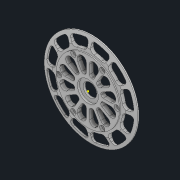
# Autodesk Inventor part: taiko_01
Saved by Autodesk Inventor 2022 (Build 260153000, 153)
## iProperties
Created: 2024-06-02
Part Number: taiko_01
Material: 一般
Document SubType Name: Modeling
Designer: gisen
Density: 1 g/cm^3
Appearance: 既定
Author: gisen
Autodesk Inventor part; units mm, degrees
ref_plane "YZ Plane" through (0, 0, 0) normal (1, 0, 0) x (0, 1, 0)
ref_plane "XZ Plane" through (0, 0, 0) normal (0, 1, 0) x (-1, 0, 0)
ref_plane "XY Plane" through (0, 0, 0) normal (0, 0, 1) x (1, 0, 0)
sketch "スケッチ1" plane through (0, 0, 0) normal (0, 0, 1) x (1, 0, 0)
  circle A0 centre (0, 0) radius 45
  circle A1 centre (0, 0) radius 6.5
  dimension "d0" = 90
  dimension "d9" = 13
  constraints: 2 centre point, 2 coincident
  measures "d0" diameter of A0
  measures "d9" diameter of A1
extrude "押し出し1" add sketch "スケッチ1" along normal blind 4
sketch "スケッチ2" plane through (0, 0, 4) normal (0, 0, 1) x (1, 0, 0)
  circle A0 centre (0, 0) radius 45 projected
  circle A1 centre (0, 0) radius 30.4
  dimension "d3" = 60.8
  constraints: 1 centre point, 1 coincident
  measures "d3" diameter of A1
extrude "押し出し2" cut sketch "スケッチ2" against normal blind 1
chamfer "面取り1" distance 2 distance2 10 1 edges at (-45, 0, 3) measured on face at (39.7326, -21.1262, 2)
sketch "スケッチ3" plane through (0, 0, 4) normal (0, 0, 1) x (1, 0, 0)
  circle A0 centre (0, 0) radius 10.05
  dimension "d10" = 20.1
  constraints: 1 centre point, 1 coincident
  measures "d10" diameter of A0
extrude "押し出し3" cut sketch "スケッチ3" against normal blind 2
sketch "スケッチ4" plane through (0, 0, 4) normal (0, 0, 1) x (1, 0, 0)
  circle A0 centre (0, 0) radius 45 construction
  circle A1 centre (0, 0) radius 30.4 construction
  circle A2 centre (0, 0) radius 10.05 construction
  circle A3 centre (0, 0) radius 13.05 construction
  circle A4 centre (0, 0) radius 42 construction
  circle A5 centre (0, 0) radius 32.5 construction
  line L0 (0, 0) -> (-45, 0) construction
  circle A6 centre (0, 0) radius 27.75 construction
  circle A7 centre (-27.75, 0) radius 4 construction
  line L1 (0, -1.5) -> (-45, -1.5) construction
  line L2 (-45, -1.5) -> (-45, 1.5) construction
  line L3 (-45, 1.5) -> (0, 1.5) construction
  line L4 (0, 1.5) -> (0, -1.5) construction
  circle A8 centre (-27.75, 0) radius 1.25
  line L5 (0.75, -1.299) -> (-38.2211, -23.799) construction
  line L6 (-39.7211, -21.201) -> (-0.75, 1.299) construction
  line L7 (1.299, -0.75) -> (-21.201, -39.7211) construction
  line L8 (-23.799, -38.2211) -> (-1.299, 0.75) construction
  line L9 (1.5, 0) -> (1.5, -45) construction
  line L10 (-1.5, -45) -> (-1.5, 0) construction
  line L11 (1.299, 0.75) -> (23.799, -38.2211) construction
  line L12 (21.201, -39.7211) -> (-1.299, -0.75) construction
  line L13 (0.75, 1.299) -> (39.7211, -21.201) construction
  line L14 (38.2211, -23.799) -> (-0.75, -1.299) construction
  line L15 (0, 1.5) -> (45, 1.5) construction
  line L16 (45, -1.5) -> (0, -1.5) construction
  line L17 (-0.75, 1.299) -> (38.2211, 23.799) construction
  line L18 (39.7211, 21.201) -> (0.75, -1.299) construction
  line L19 (-1.299, 0.75) -> (21.201, 39.7211) construction
  line L20 (23.799, 38.2211) -> (1.299, -0.75) construction
  line L21 (-1.5, 0) -> (-1.5, 45) construction
  line L22 (1.5, 45) -> (1.5, 0) construction
  line L23 (-1.299, -0.75) -> (-23.799, 38.2211) construction
  line L24 (-21.201, 39.7211) -> (1.299, 0.75) construction
  line L25 (-0.75, -1.299) -> (-39.7211, 21.201) construction
  line L26 (-38.2211, 23.799) -> (0.75, 1.299) construction
  circle A9 centre (-13.875, -24.0322) radius 4 construction
  circle A10 centre (-13.875, -24.0322) radius 1.25
  circle A11 centre (13.875, -24.0322) radius 4 construction
  circle A12 centre (13.875, -24.0322) radius 1.25
  circle A13 centre (27.75, 0) radius 4 construction
  circle A14 centre (27.75, 0) radius 1.25
  circle A15 centre (13.875, 24.0322) radius 4 construction
  circle A16 centre (13.875, 24.0322) radius 1.25
  circle A17 centre (-13.875, 24.0322) radius 4 construction
  circle A18 centre (-13.875, 24.0322) radius 1.25
  arc A19 (-12.9635, -1.5) -> (-11.9767, -5.1827) centre (0, 0) ccw
  arc A20 (-10.4767, -7.7808) -> (-7.7808, -10.4767) centre (0, 0) ccw
  arc A21 (-23.2471, -15.1538) -> (-17.1859, -21.7877) centre (0, 0) ccw
  arc A22 (-27.4617, -3.9896) -> (-24.7471, -12.5557) centre (0, 0) ccw
  arc A23 (-27.3658, -17.5317) -> (-17.5317, -27.3658) centre (0, 0) ccw
  arc A24 (-32.4654, -1.5) -> (-28.8658, -14.9336) centre (0, 0) ccw
  arc A25 (-27.4617, -3.9896) -> (-24.0419, -1.5) centre (-27.75, 0) ccw
  arc A26 (-13.32, -20.0709) -> (-17.1859, -21.7877) centre (-13.875, -24.0322) ccw
  arc A27 (-41.9732, -1.5) -> (-37.0999, -19.6876) centre (0, 0) ccw
  arc A28 (-35.5999, -22.2856) -> (-22.2856, -35.5999) centre (0, 0) ccw
  line L27 (-7.7808, -10.4767) -> (-13.32, -20.0709)
  line L28 (-17.5317, -27.3658) -> (-22.2856, -35.5999)
  line L29 (-27.3658, -17.5317) -> (-35.5999, -22.2856)
  line L30 (-10.4767, -7.7808) -> (-23.2471, -15.1538)
  line L31 (-11.9767, -5.1827) -> (-24.7471, -12.5557)
  line L32 (-28.8658, -14.9336) -> (-37.0999, -19.6876)
  line L33 (-12.9635, -1.5) -> (-24.0419, -1.5)
  line L34 (-32.4654, -1.5) -> (-41.9732, -1.5)
  line L35 (5.1827, -11.9767) -> (10.7219, -21.5709)
  arc A29 (10.7219, -21.5709) -> (10.2758, -25.7773) centre (13.875, -24.0322) ccw
  arc A30 (1.5, -27.7094) -> (10.2758, -25.7773) centre (0, 0) ccw
  arc A31 (1.5, -12.9635) -> (5.1827, -11.9767) centre (0, 0) ccw
  line L36 (1.5, -12.9635) -> (1.5, -27.7094)
  line L37 (-1.5, -12.9635) -> (-1.5, -27.7094)
  arc A32 (-10.2758, -25.7773) -> (-1.5, -27.7094) centre (0, 0) ccw
  arc A33 (-5.1827, -11.9767) -> (-1.5, -12.9635) centre (0, 0) ccw
  line L38 (-5.1827, -11.9767) -> (-10.7219, -21.5709)
  arc A34 (-10.2758, -25.7773) -> (-10.7219, -21.5709) centre (-13.875, -24.0322) ccw
  arc A35 (-14.9336, -28.8658) -> (-1.5, -32.4654) centre (0, 0) ccw
  line L39 (-14.9336, -28.8658) -> (-19.6876, -37.0999)
  arc A36 (-19.6876, -37.0999) -> (-1.5, -41.9732) centre (0, 0) ccw
  line L40 (-1.5, -32.4654) -> (-1.5, -41.9732)
  line L41 (14.9336, -28.8658) -> (19.6876, -37.0999)
  arc A37 (1.5, -41.9732) -> (19.6876, -37.0999) centre (0, 0) ccw
  arc A38 (1.5, -32.4654) -> (14.9336, -28.8658) centre (0, 0) ccw
  line L42 (1.5, -32.4654) -> (1.5, -41.9732)
  line L43 (12.9635, -1.5) -> (24.0419, -1.5)
  arc A39 (24.0419, -1.5) -> (27.4617, -3.9896) centre (27.75, 0) ccw
  arc A40 (24.7471, -12.5557) -> (27.4617, -3.9896) centre (0, 0) ccw
  arc A41 (11.9767, -5.1827) -> (12.9635, -1.5) centre (0, 0) ccw
  line L44 (11.9767, -5.1827) -> (24.7471, -12.5557)
  line L45 (10.4767, -7.7808) -> (23.2471, -15.1538)
  arc A42 (17.1859, -21.7877) -> (23.2471, -15.1538) centre (0, 0) ccw
  arc A43 (7.7808, -10.4767) -> (10.4767, -7.7808) centre (0, 0) ccw
  line L46 (7.7808, -10.4767) -> (13.32, -20.0709)
  arc A44 (17.1859, -21.7877) -> (13.32, -20.0709) centre (13.875, -24.0322) ccw
  arc A45 (17.5317, -27.3658) -> (27.3658, -17.5317) centre (0, 0) ccw
  line L47 (17.5317, -27.3658) -> (22.2856, -35.5999)
  arc A46 (22.2856, -35.5999) -> (35.5999, -22.2856) centre (0, 0) ccw
  line L48 (27.3658, -17.5317) -> (35.5999, -22.2856)
  line L49 (32.4654, -1.5) -> (41.9732, -1.5)
  arc A47 (37.0999, -19.6876) -> (41.9732, -1.5) centre (0, 0) ccw
  arc A48 (28.8658, -14.9336) -> (32.4654, -1.5) centre (0, 0) ccw
  line L50 (28.8658, -14.9336) -> (37.0999, -19.6876)
  line L51 (7.7808, 10.4767) -> (13.32, 20.0709)
  arc A49 (13.32, 20.0709) -> (17.1859, 21.7877) centre (13.875, 24.0322) ccw
  arc A50 (23.2471, 15.1538) -> (17.1859, 21.7877) centre (0, 0) ccw
  arc A51 (10.4767, 7.7808) -> (7.7808, 10.4767) centre (0, 0) ccw
  line L52 (10.4767, 7.7808) -> (23.2471, 15.1538)
  line L53 (11.9767, 5.1827) -> (24.7471, 12.5557)
  arc A52 (27.4617, 3.9896) -> (24.7471, 12.5557) centre (0, 0) ccw
  arc A53 (12.9635, 1.5) -> (11.9767, 5.1827) centre (0, 0) ccw
  line L54 (12.9635, 1.5) -> (24.0419, 1.5)
  arc A54 (27.4617, 3.9896) -> (24.0419, 1.5) centre (27.75, 0) ccw
  arc A55 (32.4654, 1.5) -> (28.8658, 14.9336) centre (0, 0) ccw
  line L55 (32.4654, 1.5) -> (41.9732, 1.5)
  arc A56 (41.9732, 1.5) -> (37.0999, 19.6876) centre (0, 0) ccw
  line L56 (28.8658, 14.9336) -> (37.0999, 19.6876)
  line L57 (17.5317, 27.3658) -> (22.2856, 35.5999)
  arc A57 (35.5999, 22.2856) -> (22.2856, 35.5999) centre (0, 0) ccw
  arc A58 (27.3658, 17.5317) -> (17.5317, 27.3658) centre (0, 0) ccw
  line L58 (27.3658, 17.5317) -> (35.5999, 22.2856)
  line L59 (-5.1827, 11.9767) -> (-10.7219, 21.5709)
  arc A59 (-10.7219, 21.5709) -> (-10.2758, 25.7773) centre (-13.875, 24.0322) ccw
  arc A60 (-1.5, 27.7094) -> (-10.2758, 25.7773) centre (0, 0) ccw
  arc A61 (-1.5, 12.9635) -> (-5.1827, 11.9767) centre (0, 0) ccw
  line L60 (-1.5, 12.9635) -> (-1.5, 27.7094)
  line L61 (1.5, 12.9635) -> (1.5, 27.7094)
  arc A62 (10.2758, 25.7773) -> (1.5, 27.7094) centre (0, 0) ccw
  arc A63 (5.1827, 11.9767) -> (1.5, 12.9635) centre (0, 0) ccw
  line L62 (5.1827, 11.9767) -> (10.7219, 21.5709)
  arc A64 (10.2758, 25.7773) -> (10.7219, 21.5709) centre (13.875, 24.0322) ccw
  arc A65 (14.9336, 28.8658) -> (1.5, 32.4654) centre (0, 0) ccw
  line L63 (14.9336, 28.8658) -> (19.6876, 37.0999)
  arc A66 (19.6876, 37.0999) -> (1.5, 41.9732) centre (0, 0) ccw
  line L64 (1.5, 32.4654) -> (1.5, 41.9732)
  line L65 (-14.9336, 28.8658) -> (-19.6876, 37.0999)
  arc A67 (-1.5, 41.9732) -> (-19.6876, 37.0999) centre (0, 0) ccw
  arc A68 (-1.5, 32.4654) -> (-14.9336, 28.8658) centre (0, 0) ccw
  line L66 (-1.5, 32.4654) -> (-1.5, 41.9732)
  line L67 (-12.9635, 1.5) -> (-24.0419, 1.5)
  arc A69 (-24.0419, 1.5) -> (-27.4617, 3.9896) centre (-27.75, 0) ccw
  arc A70 (-24.7471, 12.5557) -> (-27.4617, 3.9896) centre (0, 0) ccw
  arc A71 (-11.9767, 5.1827) -> (-12.9635, 1.5) centre (0, 0) ccw
  line L68 (-11.9767, 5.1827) -> (-24.7471, 12.5557)
  line L69 (-10.4767, 7.7808) -> (-23.2471, 15.1538)
  arc A72 (-17.1859, 21.7877) -> (-23.2471, 15.1538) centre (0, 0) ccw
  arc A73 (-7.7808, 10.4767) -> (-10.4767, 7.7808) centre (0, 0) ccw
  line L70 (-7.7808, 10.4767) -> (-13.32, 20.0709)
  arc A74 (-17.1859, 21.7877) -> (-13.32, 20.0709) centre (-13.875, 24.0322) ccw
  arc A75 (-17.5317, 27.3658) -> (-27.3658, 17.5317) centre (0, 0) ccw
  line L71 (-17.5317, 27.3658) -> (-22.2856, 35.5999)
  arc A76 (-22.2856, 35.5999) -> (-35.5999, 22.2856) centre (0, 0) ccw
  line L72 (-27.3658, 17.5317) -> (-35.5999, 22.2856)
  line L73 (-32.4654, 1.5) -> (-41.9732, 1.5)
  arc A77 (-37.0999, 19.6876) -> (-41.9732, 1.5) centre (0, 0) ccw
  arc A78 (-28.8658, 14.9336) -> (-32.4654, 1.5) centre (0, 0) ccw
  line L74 (-28.8658, 14.9336) -> (-37.0999, 19.6876)
  circle A79 centre (-27.75, 0) radius 2.5 construction
  dimension "d14" = 3
  dimension "d15" = 3
  dimension "d16" = 65
  dimension "d17" = 8
  dimension "d18" = 55.5
  dimension "d19" = 3
  dimension "d20" = 2.5
  dimension "d23" = 360
  dimension "d27" = 360
  dimension "d31" = 360
  dimension "d42" = 5
  constraints: 150 end point, 141 point on circle, 77 centre point, 57 coincident, 17 point on line, 6 collinear, 3 parallel, 2 horizontal, 2 midpoint, 1 horizontal alignment, 1 perpendicular, 376 other
  measures "d15" radial gap between concentric circles of A3 A2
  measures "d16" diameter of A5
  measures "d17" diameter of A7
  measures "d18" diameter of A6
  measures "d19" distance between parallel lines of L3 L1
  measures "d20" diameter of A8
  measures "d42" diameter of A79
extrude "押し出し4" cut sketch "スケッチ4" against normal through all
fillet "フィレット1" radius 4 24 edges at (1.5, -32.4654, 1.5) (14.9336, -28.8658, 1.5) (17.5317, -27.3658, 1.5) (27.3658, -17.5317, 1.5) (28.8658, -14.9336, 1.5) (32.4654, -1.5, 1.5) (32.4654, 1.5, 1.5) (28.8658, 14.9336, 1.5) (27.3658, 17.5317, 1.5) (17.5317, 27.3658, 1.5) (14.9336, 28.8658, 1.5) (1.5, 32.4654, 1.5) (-1.5, 32.4654, 1.5) (-14.9336, 28.8658, 1.5) (-17.5317, 27.3658, 1.5) (-27.3658, 17.5317, 1.5) (-28.8658, 14.9336, 1.5) (-32.4654, 1.5, 1.5) (-32.4654, -1.5, 1.5) (-28.8658, -14.9336, 1.5) (-27.3658, -17.5317, 1.5) (-17.5317, -27.3658, 1.5) (-14.9336, -28.8658, 1.5) (-1.5, -32.4654, 1.5)
fillet "フィレット2" radius 4 36 edges at (10.2758, -25.7773, 2) (10.7219, -21.5709, 2) (1.5, -27.7094, 2) (13.32, -20.0709, 2) (17.1859, -21.7877, 2) (23.2471, -15.1538, 2) (24.7471, -12.5557, 2) (27.4617, -3.9896, 2) (24.0419, -1.5, 2) (24.0419, 1.5, 2) (27.4617, 3.9896, 2) (24.7471, 12.5557, 2) (23.2471, 15.1538, 2) (13.32, 20.0709, 2) (17.1859, 21.7877, 2) (10.7219, 21.5709, 2) (10.2758, 25.7773, 2) (1.5, 27.7094, 2) (-1.5, 27.7094, 2) (-10.2758, 25.7773, 2) (-10.7219, 21.5709, 2) (-13.32, 20.0709, 2) (-17.1859, 21.7877, 2) (-23.2471, 15.1538, 2) (-24.7471, 12.5557, 2) (-27.4617, 3.9896, 2) (-24.0419, 1.5, 2) (-24.0419, -1.5, 2) (-27.4617, -3.9896, 2) (-24.7471, -12.5557, 2) (-23.2471, -15.1538, 2) (-17.1859, -21.7877, 2) (-13.32, -20.0709, 2) (-10.7219, -21.5709, 2) (-10.2758, -25.7773, 2) (-1.5, -27.7094, 2)
fillet "フィレット3" radius 2 24 edges at (1.5, -12.9635, 2) (5.1827, -11.9767, 2) (7.7808, -10.4767, 2) (10.4767, -7.7808, 2) (11.9767, -5.1827, 2) (12.9635, -1.5, 2) (12.9635, 1.5, 2) (11.9767, 5.1827, 2) (10.4767, 7.7808, 2) (7.7808, 10.4767, 2) (5.1827, 11.9767, 2) (1.5, 12.9635, 2) (-1.5, 12.9635, 2) (-5.1827, 11.9767, 2) (-7.7808, 10.4767, 2) (-10.4767, 7.7808, 2) (-11.9767, 5.1827, 2) (-12.9635, 1.5, 2) (-12.9635, -1.5, 2) (-11.9767, -5.1827, 2) (-10.4767, -7.7808, 2) (-7.7808, -10.4767, 2) (-5.1827, -11.9767, 2) (-1.5, -12.9635, 2)
fillet "フィレット4" radius 3 24 edges at (-22.2856, 35.5999, 0.8) (-35.5999, 22.2856, 0.8) (-37.0999, 19.6876, 0.8) (-41.9732, 1.5, 0.8) (-41.9732, -1.5, 0.8) (-37.0999, -19.6876, 0.8) (-35.5999, -22.2856, 0.8) (-22.2856, -35.5999, 0.8) (-19.6876, -37.0999, 0.8) (-1.5, -41.9732, 0.8) (1.5, -41.9732, 0.8) (19.6876, -37.0999, 0.8) (35.5999, -22.2856, 0.8) (22.2856, -35.5999, 0.8) (37.0999, -19.6876, 0.8) (41.9732, -1.5, 0.8) (41.9732, 1.5, 0.8) (37.0999, 19.6876, 0.8) (35.5999, 22.2856, 0.8) (22.2856, 35.5999, 0.8) (19.6876, 37.0999, 0.8) (1.5, 41.9732, 0.8) (-1.5, 41.9732, 0.8) (-19.6876, 37.0999, 0.8)
sketch "スケッチ5" plane through (0, 0, 4) normal (0, 0, 1) x (1, 0, 0)
  circle A0 centre (13.875, 24.0322) radius 1.25 construction
  circle A1 centre (-13.875, 24.0322) radius 1.25 construction
  circle A2 centre (-27.75, 0) radius 1.25 construction
  circle A3 centre (-13.875, -24.0322) radius 1.25 construction
  circle A4 centre (13.875, -24.0322) radius 1.25 construction
  circle A5 centre (27.75, 0) radius 1.25 construction
  circle A6 centre (13.875, 24.0322) radius 2.55
  circle A7 centre (-13.875, 24.0322) radius 2.55
  circle A8 centre (-27.75, 0) radius 2.55
  circle A9 centre (-13.875, -24.0322) radius 2.55
  circle A10 centre (13.875, -24.0322) radius 2.55
  circle A11 centre (27.75, 0) radius 2.55
  point P0 (0, 0)
  dimension "d39" = 5.1
  constraints: 6 centre point, 6 coincident, 5 equal radius
  measures "d39" diameter of A6
extrude "押し出し5" cut sketch "スケッチ5" against normal blind 2
sketch "スケッチ6" plane through (0, 0, 4) normal (0, 0, 1) x (1, 0, 0)
  point P0 (0, 0)
